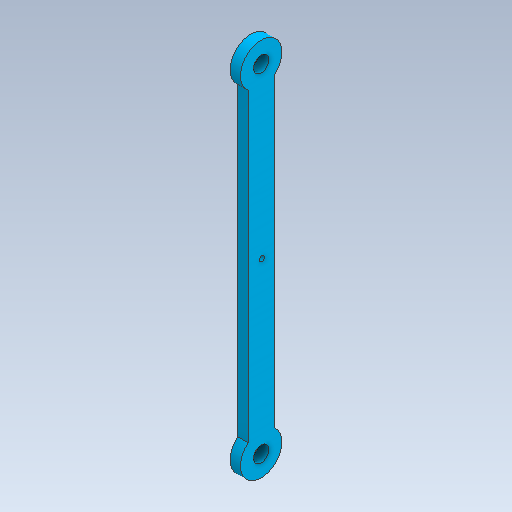
# Autodesk Inventor part: Part3
Saved by Autodesk Inventor 2020 (Build 240168000, 168)
## iProperties
Created: 2022-04-26
Part Number: Part3
Material: Generic
Document SubType Name: Modeling
Designer: Manish
Density: 1 g/cm^3
Appearance: Default
Mass: 746.783 g
Surface Area: 1104.71 cm^2
Volume: 746.783 cm^3
Author: Manish
Autodesk Inventor part; units mm, degrees
ref_plane "YZ Plane" through (0, 0, 0) normal (1, 0, 0) x (0, 1, 0)
ref_plane "XZ Plane" through (0, 0, 0) normal (0, 1, 0) x (-1, 0, 0)
ref_plane "XY Plane" through (0, 0, 0) normal (0, 0, 1) x (1, 0, 0)
sketch "Sketch1" plane through (0, 0, 0) normal (1, 0, 0) x (0, 1, 0)
  line L0 (300, 25) -> (-300, 25)
  line L1 (-300, 25) -> (-300, -25)
  line L2 (-300, -25) -> (300, -25)
  line L3 (300, -25) -> (300, 25)
  circle A0 centre (-325, 0) radius 40
  circle A1 centre (-325, 0) radius 15
  circle A2 centre (0, -1.3263) radius 5
  circle A3 centre (325, 0) radius 15
  circle A4 centre (325, 0) radius 40
  point P0 (0, 0)
  point P1 (-293.775, 25)
  point P2 (-293.775, -25)
  point P3 (293.775, -25)
  point P4 (293.775, 25)
  dimension "d0" = 600
  dimension "d1" = 50
  dimension "d2" = 25
  dimension "d3" = 300
  dimension "d4" = 30
  dimension "d5" = 25
  dimension "d6" = 80
  dimension "d11" = 10
  dimension "d14" = 0
  dimension "d15" = 30
  dimension "d16" = 80
  dimension "d17" = 25
  constraints: 8 end point, 5 centre point, 2 coincident, 2 parallel, 1 horizontal, 1 perpendicular
  measures "d0" distance of L2.end L1.end
  measures "d1" distance of L1.end L0.end
  measures "d2" distance from line of point (0, 0) L0
  measures "d3" distance from line of point (0, 0) L3
  measures "d4" diameter of A1
  measures "d5" distance from line of L1 A0.centre
  measures "d6" diameter of A0
  measures "d11" diameter of A2
  measures "d14" horizontal distance of point (0, 0) A2.centre
  measures "d15" diameter of A3
  measures "d16" diameter of A4
  measures "d17" distance from line of L3 A3.centre
extrude "Extrusion1" add sketch "Sketch1" along normal blind 20
body "Solid1"
